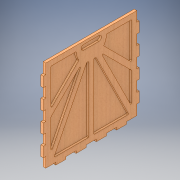
# Autodesk Inventor part: SizingCrateMinorSide
Saved by Autodesk Inventor 2017.3 (Build 213256000, 256)
## iProperties
Created: 2019-04-26
Part Number: SizingCrateMinorSide
Material: Wood (Cherry)
Document SubType Name: Modeling
Designer: guberti
Density: 0.63 g/cm^3
Appearance: Cherry - Natural Low Gloss
Author: guberti
Autodesk Inventor part; units mm, degrees
ref_plane "YZ Plane" through (0, 0, 0) normal (1, 0, 0) x (0, 1, 0)
ref_plane "XZ Plane" through (0, 0, 0) normal (0, 1, 0) x (-1, 0, 0)
ref_plane "XY Plane" through (0, 0, 0) normal (0, 0, 1) x (1, 0, 0)
sketch "Sketch1" plane through (0, 0, 0) normal (1, 0, 0) x (0, 1, 0)
  line L0 (0, -50.8) -> (-11.9062, -50.8)
  line L1 (-11.9062, -50.8) -> (-11.9063, -101.6)
  line L2 (-11.9063, -101.6) -> (0, -101.6)
  line L3 (0, -101.6) -> (0, -152.4)
  line L4 (0, -152.4) -> (-11.9063, -152.4)
  line L5 (-11.9063, -152.4) -> (-11.9063, -203.2)
  line L6 (-11.9063, -203.2) -> (0, -203.2)
  line L7 (0, 0) -> (228.6, -228.6) construction
  line L8 (0, 0) -> (323.2892, 0) construction
  line L9 (50.8, 0) -> (50.8, 11.9062)
  line L10 (50.8, 11.9062) -> (101.6, 11.9062)
  line L11 (101.6, 11.9062) -> (101.6, 0)
  line L12 (101.6, 0) -> (152.4, 0)
  line L13 (152.4, 0) -> (152.4, 11.9062)
  line L14 (152.4, 11.9062) -> (203.2, 11.9062)
  line L15 (203.2, 11.9062) -> (203.2, 0)
  line L16 (50.8, 0) -> (0, 0)
  line L17 (0, 0) -> (0, -50.8)
  line L18 (228.6, -228.6) -> (0, -228.6) construction
  line L19 (203.2, 0) -> (254, 0)
  line L20 (254, 0) -> (254, 11.9062)
  line L21 (254, 11.9062) -> (304.8, 11.9062)
  line L22 (304.8, 11.9062) -> (304.8, 0)
  line L23 (304.8, 0) -> (355.6, 0)
  line L24 (355.6, 0) -> (355.6, 11.9062)
  line L25 (355.6, 11.9062) -> (406.4, 11.9062)
  line L26 (406.4, 11.9062) -> (406.4, 0)
  line L27 (406.4, 0) -> (457.2, 0)
  line L28 (0, -406.4) -> (-11.9062, -406.4)
  line L29 (-11.9062, -406.4) -> (-11.9063, -355.6)
  line L30 (-11.9063, -355.6) -> (0, -355.6)
  line L31 (0, -355.6) -> (0, -304.8)
  line L32 (0, -304.8) -> (-11.9063, -304.8)
  line L33 (-11.9063, -304.8) -> (-11.9063, -254)
  line L34 (-11.9063, -254) -> (0, -254)
  line L35 (50.8, -457.2) -> (50.8, -469.1062)
  line L36 (50.8, -469.1062) -> (101.6, -469.1062)
  line L37 (101.6, -469.1062) -> (101.6, -457.2)
  line L38 (101.6, -457.2) -> (152.4, -457.2)
  line L39 (152.4, -457.2) -> (152.4, -469.1062)
  line L40 (152.4, -469.1062) -> (203.2, -469.1062)
  line L41 (203.2, -469.1062) -> (203.2, -457.2)
  line L42 (50.8, -457.2) -> (0, -457.2)
  line L43 (0, -457.2) -> (0, -406.4)
  line L44 (203.2, -457.2) -> (254, -457.2)
  line L45 (254, -457.2) -> (254, -469.1062)
  line L46 (254, -469.1062) -> (304.8, -469.1062)
  line L47 (304.8, -469.1062) -> (304.8, -457.2)
  line L48 (304.8, -457.2) -> (355.6, -457.2)
  line L49 (355.6, -457.2) -> (355.6, -469.1062)
  line L50 (355.6, -469.1062) -> (406.4, -469.1062)
  line L51 (406.4, -469.1062) -> (406.4, -457.2)
  line L52 (406.4, -457.2) -> (457.2, -457.2)
  line L53 (0, -203.2) -> (0, -254)
  line L54 (457.2, 0) -> (457.2, -457.2)
  dimension "thickness" = 11.9062
  dimension "toothwidth" = 50.8
  dimension "d8" = 323.2892
  dimension "d9" = 45
  dimension "d10" = 50.8
  dimension "d11" = 228.6
  constraints: 110 end point, 34 symmetric about line, 13 equal length, 12 point on line, 6 perpendicular, 4 horizontal, 4 vertical, 2 parallel
  measures "thickness" distance of L0.start L0.end
  measures "toothwidth" distance of L7.start L0.start
  measures "d8" distance of L7.start L7.end
  measures "d9" angle of L7 L8
  measures "d10" distance of L0.end L1.end
  measures "d11" distance of L7.end L18.end
extrude "Extrusion1" add sketch "Sketch1" along normal blind 12.7
sketch "Sketch2" plane through (12.7, 0, 0) normal (1, 0, 0) x (0, 0, -1)
  line L0 (26.1937, 26.1937) -> (431.0063, 26.1937) construction
  line L1 (431.0063, 26.1937) -> (431.0063, 431.0063) construction
  line L2 (431.0063, 431.0063) -> (26.1937, 431.0063) construction
  line L3 (26.1937, 431.0063) -> (26.1937, 26.1937) construction
  line L4 (190.5, 431.0062) -> (266.7, 431.0062) construction
  line L5 (190.5, 418.3063) -> (266.7, 418.3062)
  line L6 (266.7, 443.7063) -> (190.5, 443.7063)
  arc A0 (190.5, 443.7063) -> (190.5, 418.3063) centre (190.5, 431.0062) ccw
  arc A1 (266.7, 418.3062) -> (266.7, 443.7063) centre (266.7, 431.0062) ccw
  line L7 (26.1937, 228.6) -> (228.6, 431.0062) construction
  line L8 (228.6, 431.0062) -> (26.1937, 26.1937) construction
  line L9 (431.0063, 228.6) -> (228.6, 431.0062) construction
  line L10 (431.0063, 26.1937) -> (228.6, 431.0062) construction
  line L11 (228.6, 26.1938) -> (228.6, 431.0062) construction
  line L12 (166.4918, 386.8586) -> (26.1937, 246.5605)
  line L13 (26.1937, 210.6395) -> (168.296, 352.7418)
  line L14 (206.3582, 358.1246) -> (40.3928, 26.1937)
  line L15 (26.1937, 54.5918) -> (173.4216, 349.0475)
  line L16 (241.3, 26.1937) -> (241.3, 355.872)
  line L17 (215.9, 355.872) -> (215.9, 26.1938)
  line L18 (431.0063, 54.5918) -> (283.7784, 349.0475)
  line L19 (250.8418, 358.1246) -> (416.8072, 26.1937)
  line L20 (431.0063, 246.5605) -> (290.7082, 386.8586)
  line L21 (288.904, 352.7418) -> (431.0063, 210.6395)
  line L22 (304.8, 431.0063) -> (431.0063, 431.0063)
  line L23 (431.0063, 431.0063) -> (431.0063, 246.5605)
  line L24 (431.0063, 210.6395) -> (431.0063, 54.5918)
  line L25 (416.8072, 26.1937) -> (241.3, 26.1937)
  line L26 (215.9, 26.1938) -> (40.3928, 26.1937)
  line L27 (26.1937, 54.5918) -> (26.1937, 210.6395)
  line L28 (152.4, 431.0062) -> (26.1937, 431.0063)
  line L29 (26.1937, 431.0063) -> (26.1937, 246.5605)
  arc A2 (173.4216, 349.0475) -> (168.296, 352.7418) centre (170.5591, 350.4788) ccw
  arc A3 (288.904, 352.7418) -> (283.7784, 349.0475) centre (286.6409, 350.4788) ccw
  arc A4 (290.7082, 386.8586) -> (304.8, 431.0063) centre (228.6, 431.0062) ccw
  arc A5 (241.3, 355.872) -> (250.8418, 358.1246) centre (228.6, 431.0062) ccw
  arc A6 (152.4, 431.0062) -> (166.4918, 386.8586) centre (228.6, 431.0062) ccw
  arc A7 (206.3582, 358.1246) -> (215.9, 355.872) centre (228.6, 431.0062) ccw
  line L30 (457.2, 457.2) -> (0, 457.2) projected
  line L31 (-11.9062, 406.4) -> (-11.9062, 355.6) projected
  line L32 (469.1062, 355.6) -> (469.1062, 406.4) projected
  line L33 (152.4, -11.9063) -> (203.2, -11.9063) projected
  point P0 (0, 0)
  point P1 (0, 0)
  dimension "d25" = 38.1
  dimension "d26" = 25.4
  dimension "d27" = 12.7
  dimension "d28" = 12.7
  dimension "d29" = 12.7
  dimension "d30" = 12.7
  dimension "d31" = 12.7
  dimension "d32" = 12.7
  dimension "d33" = 12.7
  dimension "d34" = 12.7
  dimension "d35" = 12.7
  dimension "d36" = 12.7
  dimension "d37" = 3.2004
  dimension "d38" = 3.2004
  dimension "d39" = 76.2
  dimension "d40" = 76.2
  dimension "d41" = 76.2
  dimension "d42" = 76.2
  dimension "d44" = 26.1938
  dimension "border" = 38.1
  dimension "d46" = 38.1
  dimension "d47" = 38.1
  constraints: 62 end point, 16 point on circle, 13 point on line, 12 parallel, 8 centre point, 8 tangent, 6 collinear, 5 midpoint, 4 perpendicular, 2 coincident, 1 horizontal, 1 vertical
  measures "d25" distance of point (228.6, 431.006) L4.end
  measures "d26" diameter of A1
  measures "d27" distance between parallel lines of L12 L7
  measures "d28" distance between parallel lines of L13 L7
  measures "d29" distance between parallel lines of L15 L8
  measures "d30" distance between parallel lines of L14 L8
  measures "d31" distance between parallel lines of L16 L11
  measures "d32" distance between parallel lines of L17 L11
  measures "d33" distance between parallel lines of L10 L18
  measures "d34" distance between parallel lines of L19 L10
  measures "d35" distance between parallel lines of L20 L9
  measures "d36" distance between parallel lines of L21 L9
  measures "d37" radius of A2
  measures "d38" radius of A3
  measures "d39" radius of A6
  measures "d40" radius of A7
  measures "d41" radius of A5
  measures "d42" radius of A4
  measures "d44" distance between parallel lines of L30 L28
  measures "border" distance between parallel lines of L31 L3
  measures "d46" distance between parallel lines of L32 L1
  measures "d47" distance between parallel lines of L33 L0
extrude "Extrusion2" cut sketch "Sketch2" against normal blind 9.525
fillet "Fillet1" radius 3.1775 20 edges at (7.9375, 431.0062, -152.4) (7.9375, 431.0063, -26.1937) (7.9375, 386.8586, -166.4918) (7.9375, 246.5605, -26.1937) (7.9375, 26.1937, -40.3928) (7.9375, 26.1938, -215.9) (7.9375, 54.5918, -26.1937) (7.9375, 210.6395, -26.1937) (7.9375, 355.872, -215.9) (7.9375, 358.1246, -206.3582) (7.9375, 355.872, -241.3) (7.9375, 358.1246, -250.8418) (7.9375, 26.1937, -241.3) (7.9375, 26.1937, -416.8072) (7.9375, 54.5918, -431.0063) (7.9375, 210.6395, -431.0063) (7.9375, 246.5605, -431.0063) (7.9375, 431.0063, -431.0063) (7.9375, 386.8586, -290.7082) (7.9375, 431.0063, -304.8)
equation "\"d10\" = toothwidth"
equation "\"d28\" = d27"
equation "\"d29\" = d27"
equation "\"d30\" = d27"
equation "\"d31\" = d27"
equation "\"d32\" = d27"
equation "\"d33\" = d27"
equation "\"d34\" = d27"
equation "\"d35\" = d27"
equation "\"d36\" = d27"
equation "\"d38\" = d37"
equation "\"d40\" = d39"
equation "\"d41\" = d39"
equation "\"d42\" = d39"
equation "\"d44\" = border - thickness"
equation "\"d47\" = border"
body "Solid1"
